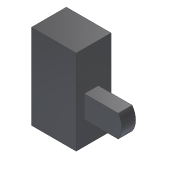
# Autodesk Inventor part: power_switch
Saved by Autodesk Inventor 2014 (Build 180170000, 170)
## iProperties
Created: 2013-06-26
Part Number: power_switch
Document SubType Name: Modeling
Designer: Administrator
Density: 1 g/cm^3
Material: Generic
Appearance: Smooth - Medium Gray
Author: Administrator
Autodesk Inventor part; units mm, degrees
ref_plane "YZ Plane" through (0, 0, 0) normal (1, 0, 0) x (0, 1, 0)
ref_plane "XZ Plane" through (0, 0, 0) normal (0, 1, 0) x (-1, 0, 0)
ref_plane "XY Plane" through (0, 0, 0) normal (0, 0, 1) x (1, 0, 0)
sketch "Sketch1" plane through (0, 0, 0) normal (0, 0, 1) x (1, 0, 0)
  line L0 (0, 0) -> (10.16, 0)
  line L1 (10.16, 0) -> (10.16, 19.304)
  line L2 (10.16, 19.304) -> (0, 19.304)
  line L3 (0, 19.304) -> (0, 0)
  dimension "d0" = 10.16
  dimension "d1" = 19.304
  constraints: 8 end point
  measures "d0" distance between parallel lines of L1 L3
  measures "d1" distance of L2.end L0.start
extrude "Extrusion1" add sketch "Sketch1" along normal blind 7.9248
sketch "Sketch2" plane through (10.16, 0, 0) normal (1, 0, 0) x (0, 0, -1)
  line L0 (0, 0) -> (-7.9248, 0) projected
  line L1 (0, 0) -> (0, 19.304) projected
  line L2 (0, 19.304) -> (-7.9248, 19.304) projected
  line L3 (-2.921, 10.414) -> (-6.096, 10.414)
  line L4 (-6.096, 10.414) -> (-6.096, 5.334)
  line L5 (-6.096, 5.334) -> (-2.921, 5.334)
  line L6 (-2.921, 5.334) -> (-2.921, 10.414)
  line L7 (-6.096, 10.414) -> (-6.096, 13.97)
  line L8 (-6.096, 13.97) -> (-2.921, 13.97)
  line L9 (-2.921, 13.97) -> (-2.921, 10.414)
  dimension "d5" = 5.08
  dimension "d6" = 3.175
  dimension "d9" = 2.921
  dimension "d10" = 3.556
  dimension "d11" = 5.334
  dimension "d13" = 5.334
  constraints: 14 end point, 4 vertical, 2 horizontal
  measures "d5" distance between parallel lines of L3 L5
  measures "d6" distance of L4.end L5.end
  measures "d9" distance between parallel lines of L1 L6
  measures "d10" distance of L8.end L3.start
  measures "d11" distance between parallel lines of L0 L5
  measures "d13" distance between parallel lines of L2 L8
extrude "Extrusion2" add sketch "Sketch2" along normal blind 8.509 contours L6 L5 L4 L3
sketch "Sketch3" plane through (10.16, 5.334, 6.096) normal (0, 0, 1) x (1, 0, 0)
  line L0 (8.509, 0) -> (8.509, 5.08) projected
  line L1 (0, 5.08) -> (8.509, 5.08) projected
  line L2 (0, 0) -> (0, 5.08) projected
  line L3 (0, 0) -> (8.509, 0) projected
  arc A0 (7.7118, 0) -> (7.7118, 5.08) centre (4.064, 2.54) ccw
  point P0 (-10.16, -5.334)
  dimension "d17" = 4.445
  constraints: 2 point on circle, 2 point on line, 1 centre point, 1 tangent
  measures "d17" radius of A0
extrude "Extrusion3" cut sketch "Sketch3" against normal through all contours L3 A0 L0 | A0 L1 L0
equation "\"d11\" = d13"
body "Solid1"
